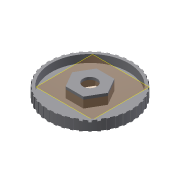
# Autodesk Inventor part: 27_Focus_Knob
Saved by Autodesk Inventor 2016 (Build 200138000, 138)
## iProperties
Created: 2017-01-03
Part Number: 27_Focus_Knob
Material: Generisch
Document SubType Name: Modeling
Designer: Bene
Density: 1 g/cm^3
Appearance: Vorgabe
Author: Bene
Autodesk Inventor part; units mm, degrees
ref_plane "YZ Plane" through (0, 0, 0) normal (1, 0, 0) x (0, 1, 0)
ref_plane "XZ Plane" through (0, 0, 0) normal (0, 1, 0) x (-1, 0, 0)
ref_plane "XY Plane" through (0, 0, 0) normal (0, 0, 1) x (1, 0, 0)
ref_plane "Arbeitsebene1" through (-4.0311, -1.75, -5) normal (0, 0, 1) x (1, 0, 0)
sketch "Skizze1" plane through (-4.0311, -1.75, -5) normal (0, 0, 1) x (1, 0, 0)
  arc A0 (6.0622, 0) -> (6.0622, 3.5) centre (3.0311, 1.75) ccw construction
  arc A1 (3.0311, -1.75) -> (6.0622, 0) centre (3.0311, 1.75) ccw construction
  arc A2 (0, 0) -> (3.0311, -1.75) centre (3.0311, 1.75) ccw construction
  arc A3 (0, 3.5) -> (0, 0) centre (3.0311, 1.75) ccw construction
  arc A4 (3.0311, 5.25) -> (0, 3.5) centre (3.0311, 1.75) ccw construction
  arc A5 (6.0622, 3.5) -> (3.0311, 5.25) centre (3.0311, 1.75) ccw construction
  circle A6 centre (3.0311, 1.75) radius 0.9894 construction
  circle A7 centre (3.0311, 1.75) radius 16
  line L0 (-2.7424, 1.75) -> (0.1443, -3.25) projected
  line L1 (8.8046, 1.75) -> (5.9178, 6.75) projected
  line L2 (5.9178, 6.75) -> (0.1443, 6.75) projected
  line L3 (0.1443, 6.75) -> (-2.7424, 1.75) projected
  line L4 (5.9178, -3.25) -> (8.8046, 1.75) projected
  line L5 (0.1443, -3.25) -> (5.9178, -3.25) projected
  line L6 (5.9178, -3.25) -> (0.1443, -3.25)
  line L7 (0.1443, -3.25) -> (-2.7424, 1.75)
  line L8 (-2.7424, 1.75) -> (0.1443, 6.75)
  line L9 (0.1443, 6.75) -> (5.9178, 6.75)
  line L10 (5.9178, 6.75) -> (8.8046, 1.75)
  line L11 (8.8046, 1.75) -> (5.9178, -3.25)
  dimension "d1" = 32
  constraints: 12 end point, 1 centre point, 1 coincident, 14 other
  measures "d1" diameter of A7
extrude "Extrusion1" add sketch "Skizze1" against normal blind 4
shell "Wandung1" thickness 1 removed faces 1 at (-8.6092, -4.1452, -5)
sketch "Skizze2" plane through (-4.0311, -1.75, -5) normal (0, 0, 1) x (1, 0, 0)
  circle A0 centre (3.0311, 1.75) radius 2.3866 construction
  line L0 (9.9593, 1.75) -> (6.4952, 7.75) projected
  line L1 (6.4952, 7.75) -> (-0.433, 7.75) projected
  line L2 (-0.433, 7.75) -> (-3.8971, 1.75) projected
  line L3 (-3.8971, 1.75) -> (-0.433, -4.25) projected
  line L4 (-0.433, -4.25) -> (6.4952, -4.25) projected
  line L5 (6.4952, -4.25) -> (9.9593, 1.75) projected
  line L6 (5.9178, 6.75) -> (8.8046, 1.75) projected
  line L7 (8.8046, 1.75) -> (5.9178, -3.25) projected
  line L8 (5.9178, -3.25) -> (0.1443, -3.25) projected
  line L9 (0.1443, -3.25) -> (-2.7424, 1.75) projected
  line L10 (-2.7424, 1.75) -> (0.1443, 6.75) projected
  line L11 (0.1443, 6.75) -> (5.9178, 6.75) projected
  circle A1 centre (3.0311, 1.75) radius 2.3866 projected
  circle A2 centre (3.0311, 1.75) radius 2.6866
  dimension "d16" = 0.3
  constraints: 1 centre point
  measures "d16" radial gap between concentric circles of A0 A2
extrude "Extrusion2" add sketch "Skizze2" along normal blind 1 contours L5 L4 L3 L2 L1 L0 | L6 L7 L8 L9 L10 L11
sketch "Skizze3" plane through (0, 0, 0) normal (0, 1, 0) x (-1, 0, 0)
  line L0 (-16, -9) -> (16, -9)
  line L1 (-15, -5) -> (16, -5)
  line L2 (-15, -5) -> (-15.3, -5)
  line L3 (-15.3, -5) -> (-15.3, -9)
  line L4 (-15.3, -9) -> (-15, -9)
  line L5 (-15, -9) -> (-15, -5)
  line L6 (2, -19.9) -> (2, -0.4294)
  line L7 (-2, -19.9) -> (-2, -0.4294)
  line L8 (0, -15.3981) -> (0, 0)
  line L9 (-15, -5) -> (-14.7, -5)
  line L10 (-14.7, -5) -> (-14.7, -9)
  line L11 (-14.7, -9) -> (-15, -9)
  line L12 (-15, -9) -> (-15, -5)
  line L13 (-15, -5) -> (-15, -9) projected
  line L14 (-15, -9) -> (17, -9) projected
  dimension "d8" = 0.3
  dimension "d11" = 0.3
  constraints: 26 end point, 4 parallel, 3 vertical, 2 horizontal, 2 perpendicular, 2 point on line, 4 other
  measures "d8" distance of L4.end L3.end
  measures "d11" distance of L10.end L11.end
extrude "Extrusion3" add sketch "Skizze3" along normal mid plane 1 contours L3 L2 L5 L0 | L5 L1 L10 L0
pattern_circular "Runde Anordnung1" count 40 over 360 about axis through (-1, 0, -5) along (0, 0, 1) of "Extrusion3"
